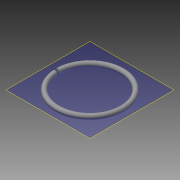
# Autodesk Inventor part: Loop
Saved by Autodesk Inventor 2013 (Build 170138000, 138)
## iProperties
Created: 2014-03-24
Part Number: Loop
Material: Generic
Document SubType Name: Modeling
Designer: jad211
Density: 1 g/cm^3
Author: jad211
Autodesk Inventor part; units mm, degrees
ref_plane "YZ Plane" through (0, 0, 0) normal (1, 0, 0) x (0, 1, 0)
ref_plane "XZ Plane" through (0, 0, 0) normal (0, 1, 0) x (-1, 0, 0)
ref_plane "XY Plane" through (0, 0, 0) normal (0, 0, 1) x (1, 0, 0)
sketch "Sketch1" plane through (0, 0, 0) normal (0, 1, 0) x (-1, 0, 0)
  circle A0 centre (20, 0) radius 1.5
  line L0 (0, -2.1) -> (0, 2.1) projected
  point P0 (0, 0)
  dimension "d0" = 3
  dimension "d3" = 20
  constraints: 1 centre point
  measures "d0" diameter of A0
  measures "d3" distance of A0.centre point (0, 0)
revolve "Revolution1" add sketch "Sketch1" angle 355 about axis through (0, 0, -10) along (0, 0, -1)
ref_plane "Work Plane1" through (0, 0, 0) normal (0, 0, -1) x (-1, 0, 0)
body "Solid1"
